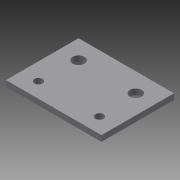
# Autodesk Inventor part: servo catch back c
Saved by Autodesk Inventor 2015 (Build 190159000, 159)
## iProperties
Created: 2015-06-24
Part Number: servo catch back c
Material: 一般
Document SubType Name: Modeling
Designer: kenta
Density: 1 g/cm^3
Appearance: 既定
Author: kenta
Autodesk Inventor part; units mm, degrees
ref_plane "YZ Plane" through (0, 0, 0) normal (1, 0, 0) x (0, 1, 0)
ref_plane "XZ Plane" through (0, 0, 0) normal (0, 1, 0) x (-1, 0, 0)
ref_plane "XY Plane" through (0, 0, 0) normal (0, 0, 1) x (1, 0, 0)
sketch "スケッチ1" plane through (0, 0, 0) normal (0, 0, 1) x (1, 0, 0)
  line L0 (-12.5, 9.5) -> (12.5, 9.5)
  line L1 (12.5, 9.5) -> (12.5, -9.5)
  line L2 (12.5, -9.5) -> (-12.5, -9.5)
  line L3 (-12.5, -9.5) -> (-12.5, 9.5)
  line L4 (-12.5, 9.5) -> (12.5, -9.5) construction
  line L5 (12.5, 9.5) -> (-12.5, -9.5) construction
  point P0 (0, 0)
  dimension "d0" = 25
  dimension "d1" = 19
  constraints: 12 end point, 2 midpoint, 2 parallel, 1 horizontal, 1 perpendicular
  measures "d0" distance of L1.end L2.end
  measures "d1" distance of L0.end L1.end
extrude "押し出し1" add sketch "スケッチ1" along normal blind 1.5
sketch "スケッチ2" plane through (0, 0, 1.5) normal (0, 0, 1) x (1, 0, 0)
  line L0 (-12.5, -9.5) -> (12.5, -9.5) projected
  line L1 (-12.5, 9.5) -> (-12.5, -9.5) projected
  line L2 (12.5, -9.5) -> (12.5, 9.5) projected
  point P0 (0, 0)
  point P1 (-8, -5.5)
  point P2 (8, -5.5)
  dimension "d4" = 4
  dimension "d5" = 4.5
  dimension "d6" = 4.5
  dimension "d7" = 4
  constraints: 1 horizontal alignment
  measures "d4" distance from line of point (-8, -5.5) L0
  measures "d5" distance from line of L1 point (-8, -5.5)
  measures "d6" distance from line of point (8, -5.5) L2
  measures "d7" distance from line of point (8, -5.5) L0
hole "穴1" at (-8, -5.5, 1.5) at (8, -5.5, 1.5) direction (0, 0, -1) diameter 2.1 end through all
sketch "スケッチ3" plane through (0, 0, 1.5) normal (0, 0, 1) x (1, 0, 0)
  line L0 (12.5, -9.5) -> (12.5, 9.5) projected
  line L1 (12.5, 9.5) -> (-12.5, 9.5) projected
  line L2 (-12.5, 9.5) -> (-12.5, -9.5) projected
  point P0 (0, 0)
  point P1 (-7.5, 4.5)
  point P2 (7.5, 4.5)
  dimension "d15" = 5
  dimension "d16" = 5
  dimension "d17" = 5
  dimension "d18" = 5
  constraints: 1 horizontal alignment
  measures "d15" distance from line of point (7.5, 4.5) L0
  measures "d16" distance from line of point (7.5, 4.5) L1
  measures "d17" distance from line of L1 point (-7.5, 4.5)
  measures "d18" distance from line of point (-7.5, 4.5) L2
hole "穴2" at (-7.5, 4.5, 1.5) at (7.5, 4.5, 1.5) direction (0, 0, -1) diameter 3.1 end through all
